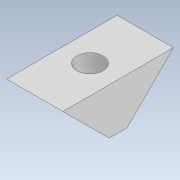
# Autodesk Inventor part: buttom_camera_fix
Saved by Autodesk Inventor 2020 (Build 240168000, 168)
## iProperties
Created: 2021-02-02
Part Number: buttom_camera_fix
Material: Generic
Document SubType Name: Modeling
Designer: DELL
Density: 1 g/cm^3
Appearance: Default
Author: DELL
Autodesk Inventor part; units mm, degrees
ref_plane "YZ Plane" through (0, 0, 0) normal (1, 0, 0) x (0, 1, 0)
ref_plane "XZ Plane" through (0, 0, 0) normal (0, 1, 0) x (-1, 0, 0)
ref_plane "XY Plane" through (0, 0, 0) normal (0, 0, 1) x (1, 0, 0)
sketch "Sketch1" plane through (0, 0, 0) normal (1, 0, 0) x (0, 1, 0)
  line L0 (0, 4.5) -> (0, -4.5)
  line L1 (0, -4.5) -> (23, -27.5)
  line L2 (23, -27.5) -> (23, 27.5)
  line L3 (23, 27.5) -> (0, 4.5)
  point P0 (0, 0)
  point P1 (0, 0)
  point P2 (23, 0)
  dimension "d0" = 45
  dimension "d1" = 55
  dimension "d2" = 23
  constraints: 8 end point, 2 midpoint, 1 coincident, 1 horizontal alignment, 1 parallel, 1 vertical
  measures "d0" angle of L0 L3
  measures "d1" distance of L1.end L2.end
  measures "d2" distance between parallel lines of L0 L2
extrude "Extrusion1" add sketch "Sketch1" along normal mid plane 28
sketch "Sketch2" plane through (-14, 23, 27.5) normal (0, 1, 0) x (1, 0, 0)
  circle A0 centre (14, 27.5) radius 6.5
  dimension "d5" = 13
  constraints: 1 centre point, 1 coincident
  measures "d5" diameter of A0
extrude "Extrusion2" cut sketch "Sketch2" against normal through all
body "Solid1"
